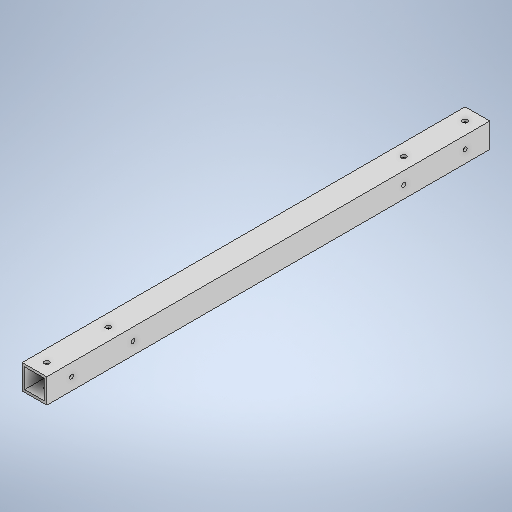
# Autodesk Inventor part: small_kaku_2020_tka
Saved by Autodesk Inventor 2025.1 (Build 291241000, 241)
## iProperties
Created: 2024-12-20
Part Number: small_kaku_2020_tka
Material: 一般
Document SubType Name: Modeling
Designer: yuki0520
Density: 1 g/cm^3
Appearance: 既定
Author: yuki0520
Autodesk Inventor part; units mm, degrees
ref_plane "YZ Plane" through (0, 0, 0) normal (1, 0, 0) x (0, 1, 0)
ref_plane "XZ Plane" through (0, 0, 0) normal (0, 1, 0) x (-1, 0, 0)
ref_plane "XY Plane" through (0, 0, 0) normal (0, 0, 1) x (1, 0, 0)
sketch "スケッチ1" plane through (0, 0, 0) normal (0, 0, 1) x (1, 0, 0)
  line L0 (10, -10) -> (-10, -10)
  line L1 (-10, -10) -> (-10, 10)
  line L2 (-10, 10) -> (10, 10)
  line L3 (10, 10) -> (10, -10)
  line L4 (10, -10) -> (-10, 10) construction
  line L5 (-10, -10) -> (10, 10) construction
  line L6 (8, 8) -> (-8, 8)
  line L7 (-8, 8) -> (-8, -8)
  line L8 (-8, -8) -> (8, -8)
  line L9 (8, -8) -> (8, 8)
  point P0 (0, 0)
  dimension "d0" = 20
  dimension "d1" = 20
  dimension "d2" = 2
  constraints: 20 end point, 4 parallel, 2 midpoint, 2 perpendicular, 1 horizontal, 3 other
  measures "d0" distance of L1.end L2.end
  measures "d1" distance of L0.end L1.end
  measures "d2" distance between parallel lines of L2 L6
extrude "押し出し1" add sketch "スケッチ1" along normal blind 360
sketch "スケッチ2" plane through (-10, 10, 0) normal (0, 1, 0) x (1, 0, 0)
  line L0 (10, 0) -> (10, -360)
  line L1 (2, -360) -> (18, -360) projected
  line L2 (20, 0) -> (0, 0) projected
  point P0 (10, -350)
  point P1 (10, -300)
  point P2 (10, -60)
  point P3 (10, -10)
  dimension "d5" = 10
  dimension "d6" = 50
  dimension "d7" = 50
  dimension "d9" = 10
  constraints: 4 point on line, 2 end point, 1 midpoint
  measures "d5" distance from line of L1 point (10, -350)
  measures "d6" distance of point (10, -300) point (10, -350)
  measures "d7" distance of point (10, -10) point (10, -60)
  measures "d9" distance from line of L2 point (10, -10)
hole "穴1" at (0, 10, 350) at (0, 10, 300) at (0, 10, 60) at (0, 10, 10) direction (0, -1, 0) diameter 4 end through all
sketch "スケッチ3" plane through (10, -10, 0) normal (1, 0, 0) x (0, 0, -1)
  line L0 (0, 10) -> (-360, 10)
  line L1 (-360, 20) -> (-360, 0) projected
  line L2 (0, 0) -> (0, 20) projected
  point P0 (-340, 10)
  point P1 (-290, 10)
  point P2 (-20, 10)
  point P3 (-70, 10)
  dimension "d17" = 20
  dimension "d18" = 50
  dimension "d19" = 20
  dimension "d20" = 50
  constraints: 4 point on line, 2 end point, 1 midpoint
  measures "d17" distance from line of L1 point (-340, 10)
  measures "d18" distance of point (-290, 10) point (-340, 10)
  measures "d19" distance from line of L2 point (-20, 10)
  measures "d20" distance of point (-20, 10) point (-70, 10)
hole "穴2" at (10, 0, 340) at (10, 0, 290) at (10, 0, 20) at (10, 0, 70) direction (-1, 0, 0) diameter 3.3 end through all
equation "\"d7\" = d6"
equation "\"d9\" = d5"
equation "\"d19\" = d17"
equation "\"d20\" = d18"
